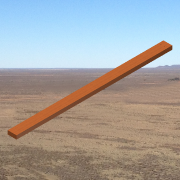
# Autodesk Inventor part: pole_EdgeRim37
Saved by Autodesk Inventor 2013 SP2 (Build 170200200, 200)
## iProperties
Created: 2013-09-03
Part Number: pole_EdgeRim37
Material: Wood (Cherry)
Document SubType Name: Modeling
Designer: Dave
Mass: 3011.12 g
Surface Area: 4583.86 cm^2
Volume: 6022.25 cm^3
Density: 0.5 g/cm^3
Author: Dave
Autodesk Inventor part; units mm, degrees
ref_plane "YZ Plane" through (0, 0, 0) normal (1, 0, 0) x (0, 1, 0)
ref_plane "XZ Plane" through (0, 0, 0) normal (0, 1, 0) x (-1, 0, 0)
ref_plane "XY Plane" through (0, 0, 0) normal (0, 0, 1) x (1, 0, 0)
sketch "Sketch1" plane through (0, 0, 0) normal (0, 0, 1) x (1, 0, 0)
  line L0 (0, 0) -> (88.9, 0)
  line L1 (88.9, 0) -> (88.9, 38.1)
  line L2 (88.9, 38.1) -> (0, 38.1)
  line L3 (0, 38.1) -> (0, 0)
  dimension "d0" = 88.9
  dimension "d1" = 38.1
  constraints: 8 end point, 2 parallel, 1 horizontal, 1 perpendicular
  measures "d0" distance of L0.start L0.end
  measures "d1" distance of L2.end L0.start
extrude "Extrusion1" add sketch "Sketch1" along normal blind 1579.88
sketch "Sketch2" plane through (0, 38.1, 0) normal (0, 1, 0) x (1, 0, 0)
  line L0 (88.9, 0) -> (0, 0) projected
  line L1 (0, 0) -> (0, -1579.88) projected
  circle A0 centre (25.4, -50.8) radius 5.7238
  circle A1 centre (63.5, -50.8) radius 5.7238
  dimension "d4" = 50.8
  dimension "d5" = 25.4
  dimension "d8" = 38.1
  constraints: 2 centre point, 1 horizontal, 2 other
  measures "d4" distance from line of A0.centre L0
  measures "d5" distance from line of L1 A0.centre
  measures "d8" distance of A0.centre A1.centre
hole "Hole1" at (25.4, 38.1, 50.8) at (63.5, 38.1, 50.8) direction (0, -1, 0) diameter 6.35 end through all
body "Solid1"
